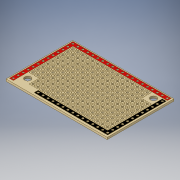
# Autodesk Inventor part: Proto Board
Saved by Autodesk Inventor 2016 (Build 200138000, 138)
## iProperties
Created: 2015-11-30
Part Number: Proto Board
Material: Generic
Document SubType Name: Modeling
Designer: Spooner
Density: 1 g/cm^3
Appearance: Beige
Author: Spooner
Autodesk Inventor part; units mm, degrees
(part 1 of 2)
ref_plane "YZ Plane" through (0, 0, 0) normal (1, 0, 0) x (0, 1, 0)
ref_plane "XZ Plane" through (0, 0, 0) normal (0, 1, 0) x (-1, 0, 0)
ref_plane "XY Plane" through (0, 0, 0) normal (0, 0, 1) x (1, 0, 0)
sketch "Sketch1" plane through (0, 0, 0) normal (0, 1, 0) x (-1, 0, 0)
  line L0 (0, 0) -> (-51.7271, 0)
  line L1 (-51.7271, 0) -> (-51.7271, -34.1376)
  line L2 (-51.7271, -34.1376) -> (0, -34.1376)
  line L3 (0, -34.1376) -> (0, 0)
  circle A0 centre (-5.3848, -5.7023) radius 1.524
  circle A1 centre (-46.3423, -29.0957) radius 1.524
  dimension "d0" = 51.7271
  dimension "d1" = 34.1376
  dimension "d2" = 3.8608
  dimension "d3" = 3.8608
  dimension "d4" = 3.5179
  dimension "d5" = 4.1783
  dimension "d6" = 3.048
  constraints: 8 end point, 2 centre point, 2 parallel, 1 equal radius, 1 horizontal, 1 perpendicular
  measures "d0" distance of L1.end L2.end
  measures "d1" distance of L2.end L0.start
  measures "d2" distance edge to line of A0 L3
  measures "d3" distance edge to line of A1 L1
  measures "d4" distance edge to line of A1 L2
  measures "d5" distance edge to line of A0 L0
  measures "d6" diameter of A0
extrude "Extrusion1" add sketch "Sketch1" along normal blind 1.016
sketch "Sketch2" plane through (0, 1.016, 0) normal (0, 1, 0) x (1, 0, 0)
  circle A0 centre (1.5494, 2.159) radius 0.508
  line L0 (0, 0) -> (51.7271, 0) projected
  line L1 (0, 34.1376) -> (0, 0) projected
  dimension "d9" = 1.016
  dimension "d10" = 1.651
  dimension "d11" = 1.0414
  constraints: 1 centre point
  measures "d9" diameter of A0
  measures "d10" distance edge to line of A0 L0
  measures "d11" distance edge to line of A0 L1
extrude "Extrusion2" cut sketch "Sketch2" against normal through all
sketch "Sketch6" plane through (0, 1.016, 0) normal (0, 1, 0) x (1, 0, 0)
  circle A0 centre (1.5494, 2.159) radius 0.508 projected
  line L0 (2.5654, 1.143) -> (0.5334, 1.143)
  line L1 (0.5334, 1.143) -> (0.5334, 3.175)
  line L2 (0.5334, 3.175) -> (2.5654, 3.175)
  line L3 (2.5654, 3.175) -> (2.5654, 1.143)
  line L4 (2.5654, 1.143) -> (0.5334, 3.175) construction
  line L5 (0.5334, 1.143) -> (2.5654, 3.175) construction
  point P0 (0, 0)
  dimension "d30" = 2.032
  constraints: 12 end point, 2 midpoint, 2 parallel, 2 perpendicular, 1 horizontal
  measures "d30" distance of L1.end L2.end
extrude "Extrusion6" add sketch "Sketch6" along normal blind 0.0254
pattern_linear "Rectangular Pattern1" count 13 spacing 2.54 along (0, 0, -1) count 20 spacing 2.54 along (1, 0, 0) of "Extrusion2", "Extrusion6"
sketch "Sketch7" plane through (0, 1.016, 0) normal (0, 1, 0) x (1, 0, 0)
  line L0 (5.6134, 3.683) -> (7.6454, 3.683) projected
  line L1 (3.0734, 8.255) -> (7.6454, 8.255)
  line L2 (7.6454, 8.255) -> (7.6454, 3.683)
  line L3 (7.6454, 3.683) -> (3.0734, 3.683)
  line L4 (3.0734, 3.683) -> (3.0734, 8.255)
  line L5 (5.1054, 3.175) -> (3.0734, 3.175) projected
  line L6 (10.6934, 1.143) -> (12.7254, 1.143) projected
  line L7 (3.0734, 3.175) -> (12.7254, 3.175)
  line L8 (12.7254, 3.175) -> (12.7254, 1.143)
  line L9 (12.7254, 1.143) -> (3.0734, 1.143)
  line L10 (3.0734, 1.143) -> (3.0734, 3.175)
  line L11 (45.7454, 31.115) -> (43.7134, 31.115) projected
  line L12 (43.7134, 31.115) -> (48.2854, 31.115)
  line L13 (48.2854, 31.115) -> (48.2854, 26.543)
  line L14 (48.2854, 26.543) -> (43.7134, 26.543)
  line L15 (43.7134, 26.543) -> (43.7134, 31.115)
  point P0 (0, 0)
  constraints: 24 end point, 6 parallel, 3 horizontal, 3 perpendicular, 2 coincident
extrude "Extrusion7" cut sketch "Sketch7" along normal blind 0.0254
sketch "Sketch8" plane through (0, 1.016, 0) normal (0, 1, 0) x (1, 0, 0)
  line L0 (3.2284, 8.3049) -> (7.6265, 8.3049)
  line L1 (7.6265, 8.3049) -> (7.6265, 3.6729)
  line L2 (7.6265, 3.6729) -> (3.2284, 3.6729)
  line L3 (3.2284, 3.6729) -> (3.2284, 8.3049)
  line L4 (3.2284, 3.1582) -> (12.6328, 3.1582)
  line L5 (12.6328, 3.1582) -> (12.6328, 1.0527)
  line L6 (12.6328, 1.0527) -> (3.2284, 1.0527)
  line L7 (3.2284, 1.0527) -> (3.2284, 3.1582)
  circle A0 centre (5.3848, 5.7023) radius 1.524
  arc A1 (6.1798, 7.0025) -> (4.5048, 6.9465) centre (5.3848, 5.7023) ccw projected
  circle A2 centre (46.3423, 29.0957) radius 1.524
  arc A3 (47.4393, 28.0378) -> (47.6879, 29.8111) centre (46.3423, 29.0957) ccw projected
  line L8 (43.7779, 31.0602) -> (48.4629, 31.0602)
  line L9 (48.4629, 31.0602) -> (48.4629, 26.515)
  line L10 (48.4629, 26.515) -> (43.7779, 26.515)
  line L11 (43.7779, 26.515) -> (43.7779, 31.0602)
  point P0 (0, 0)
  constraints: 24 end point, 6 parallel, 3 horizontal, 3 perpendicular, 1 point on line, 8 other
extrude "Extrusion8" add sketch "Sketch8" against normal up to surface (1.016 mm away)
sketch "Sketch9" plane through (0, 1.016, 0) normal (0, 1, 0) x (1, 0, 0)
  circle A0 centre (1.5494, 2.159) radius 0.508 projected
  line L0 (0.5334, 1.143) -> (2.5654, 1.143) projected
  line L1 (2.5654, 1.143) -> (2.5654, 3.175) projected
  line L2 (2.5654, 3.175) -> (0.5334, 3.175) projected
  line L3 (0.5334, 3.175) -> (0.5334, 1.143) projected
  circle A1 centre (5.3848, 5.7023) radius 1.524 projected
  circle A2 centre (46.3423, 29.0957) radius 1.524 projected
  line L4 (48.7934, 31.623) -> (48.7934, 33.655) projected
  line L5 (48.7934, 33.655) -> (50.8254, 33.655) projected
  line L6 (50.8254, 33.655) -> (50.8254, 31.623) projected
  line L7 (50.8254, 31.623) -> (48.7934, 31.623) projected
  line L8 (48.7934, 29.083) -> (48.7934, 31.115) projected
  line L9 (48.7934, 31.115) -> (50.8254, 31.115) projected
  line L10 (50.8254, 31.115) -> (50.8254, 29.083) projected
  line L11 (50.8254, 29.083) -> (48.7934, 29.083) projected
  line L12 (48.7934, 26.543) -> (48.7934, 28.575) projected
  line L13 (48.7934, 28.575) -> (50.8254, 28.575) projected
  line L14 (50.8254, 28.575) -> (50.8254, 26.543) projected
  line L15 (50.8254, 26.543) -> (48.7934, 26.543) projected
  line L16 (48.7934, 24.003) -> (48.7934, 26.035) projected
  line L17 (48.7934, 26.035) -> (50.8254, 26.035) projected
  line L18 (50.8254, 26.035) -> (50.8254, 24.003) projected
  line L19 (50.8254, 24.003) -> (48.7934, 24.003) projected
  line L20 (48.7934, 21.463) -> (48.7934, 23.495) projected
  line L21 (48.7934, 23.495) -> (50.8254, 23.495) projected
  line L22 (50.8254, 23.495) -> (50.8254, 21.463) projected
  line L23 (50.8254, 21.463) -> (48.7934, 21.463) projected
  line L24 (48.7934, 18.923) -> (48.7934, 20.955) projected
  line L25 (48.7934, 20.955) -> (50.8254, 20.955) projected
  line L26 (50.8254, 20.955) -> (50.8254, 18.923) projected
  line L27 (50.8254, 18.923) -> (48.7934, 18.923) projected
  line L28 (48.7934, 16.383) -> (48.7934, 18.415) projected
  line L29 (48.7934, 18.415) -> (50.8254, 18.415) projected
  line L30 (50.8254, 18.415) -> (50.8254, 16.383) projected
  line L31 (50.8254, 16.383) -> (48.7934, 16.383) projected
  line L32 (48.7934, 13.843) -> (48.7934, 15.875) projected
  line L33 (48.7934, 15.875) -> (50.8254, 15.875) projected
  line L34 (50.8254, 15.875) -> (50.8254, 13.843) projected
  line L35 (50.8254, 13.843) -> (48.7934, 13.843) projected
  line L36 (48.7934, 11.303) -> (48.7934, 13.335) projected
  line L37 (48.7934, 13.335) -> (50.8254, 13.335) projected
  line L38 (50.8254, 13.335) -> (50.8254, 11.303) projected
  line L39 (50.8254, 11.303) -> (48.7934, 11.303) projected
  line L40 (48.7934, 8.763) -> (48.7934, 10.795) projected
  line L41 (48.7934, 10.795) -> (50.8254, 10.795) projected
  line L42 (50.8254, 10.795) -> (50.8254, 8.763) projected
  line L43 (50.8254, 8.763) -> (48.7934, 8.763) projected
  line L44 (48.7934, 6.223) -> (48.7934, 8.255) projected
  line L45 (48.7934, 8.255) -> (50.8254, 8.255) projected
  line L46 (50.8254, 8.255) -> (50.8254, 6.223) projected
  line L47 (50.8254, 6.223) -> (48.7934, 6.223) projected
  line L48 (48.7934, 3.683) -> (48.7934, 5.715) projected
  line L49 (48.7934, 5.715) -> (50.8254, 5.715) projected
  line L50 (50.8254, 5.715) -> (50.8254, 3.683) projected
  line L51 (50.8254, 3.683) -> (48.7934, 3.683) projected
  line L52 (48.7934, 1.143) -> (48.7934, 3.175) projected
  line L53 (48.7934, 3.175) -> (50.8254, 3.175) projected
  line L54 (50.8254, 3.175) -> (50.8254, 1.143) projected
  line L55 (50.8254, 1.143) -> (48.7934, 1.143) projected
  line L56 (46.2534, 31.623) -> (46.2534, 33.655) projected
  line L57 (46.2534, 33.655) -> (48.2854, 33.655) projected
  line L58 (48.2854, 33.655) -> (48.2854, 31.623) projected
  line L59 (48.2854, 31.623) -> (46.2534, 31.623) projected
  line L60 (46.2534, 24.003) -> (46.2534, 26.035) projected
  line L61 (46.2534, 26.035) -> (48.2854, 26.035) projected
  line L62 (48.2854, 26.035) -> (48.2854, 24.003) projected
  line L63 (48.2854, 24.003) -> (46.2534, 24.003) projected
  line L64 (46.2534, 21.463) -> (46.2534, 23.495) projected
  line L65 (46.2534, 23.495) -> (48.2854, 23.495) projected
  line L66 (48.2854, 23.495) -> (48.2854, 21.463) projected
  line L67 (48.2854, 21.463) -> (46.2534, 21.463) projected
  line L68 (46.2534, 18.923) -> (46.2534, 20.955) projected
  line L69 (46.2534, 20.955) -> (48.2854, 20.955) projected
  line L70 (48.2854, 20.955) -> (48.2854, 18.923) projected
  line L71 (48.2854, 18.923) -> (46.2534, 18.923) projected
  line L72 (46.2534, 16.383) -> (46.2534, 18.415) projected
  line L73 (46.2534, 18.415) -> (48.2854, 18.415) projected
  line L74 (48.2854, 18.415) -> (48.2854, 16.383) projected
  line L75 (48.2854, 16.383) -> (46.2534, 16.383) projected
  line L76 (46.2534, 13.843) -> (46.2534, 15.875) projected
  line L77 (46.2534, 15.875) -> (48.2854, 15.875) projected
  line L78 (48.2854, 15.875) -> (48.2854, 13.843) projected
  line L79 (48.2854, 13.843) -> (46.2534, 13.843) projected
  line L80 (46.2534, 11.303) -> (46.2534, 13.335) projected
  line L81 (46.2534, 13.335) -> (48.2854, 13.335) projected
  line L82 (48.2854, 13.335) -> (48.2854, 11.303) projected
  line L83 (48.2854, 11.303) -> (46.2534, 11.303) projected
  line L84 (46.2534, 8.763) -> (46.2534, 10.795) projected
  line L85 (46.2534, 10.795) -> (48.2854, 10.795) projected
  line L86 (48.2854, 10.795) -> (48.2854, 8.763) projected
  line L87 (48.2854, 8.763) -> (46.2534, 8.763) projected
  line L88 (46.2534, 6.223) -> (46.2534, 8.255) projected
  line L89 (46.2534, 8.255) -> (48.2854, 8.255) projected
  line L90 (48.2854, 8.255) -> (48.2854, 6.223) projected
  line L91 (48.2854, 6.223) -> (46.2534, 6.223) projected
  line L92 (46.2534, 3.683) -> (46.2534, 5.715) projected
  line L93 (46.2534, 5.715) -> (48.2854, 5.715) projected
  line L94 (48.2854, 5.715) -> (48.2854, 3.683) projected
  line L95 (48.2854, 3.683) -> (46.2534, 3.683) projected
  line L96 (46.2534, 1.143) -> (46.2534, 3.175) projected
  line L97 (46.2534, 3.175) -> (48.2854, 3.175) projected
  line L98 (48.2854, 3.175) -> (48.2854, 1.143) projected
  line L99 (48.2854, 1.143) -> (46.2534, 1.143) projected
  line L100 (43.7134, 31.623) -> (43.7134, 33.655) projected
  line L101 (43.7134, 33.655) -> (45.7454, 33.655) projected
  line L102 (45.7454, 33.655) -> (45.7454, 31.623) projected
  line L103 (45.7454, 31.623) -> (43.7134, 31.623) projected
  line L104 (43.7134, 24.003) -> (43.7134, 26.035) projected
  line L105 (43.7134, 26.035) -> (45.7454, 26.035) projected
  line L106 (45.7454, 26.035) -> (45.7454, 24.003) projected
  line L107 (45.7454, 24.003) -> (43.7134, 24.003) projected
  line L108 (43.7134, 21.463) -> (43.7134, 23.495) projected
  line L109 (43.7134, 23.495) -> (45.7454, 23.495) projected
  line L110 (45.7454, 23.495) -> (45.7454, 21.463) projected
  line L111 (45.7454, 21.463) -> (43.7134, 21.463) projected
  line L112 (43.7134, 18.923) -> (43.7134, 20.955) projected
  line L113 (43.7134, 20.955) -> (45.7454, 20.955) projected
  line L114 (45.7454, 20.955) -> (45.7454, 18.923) projected
  line L115 (45.7454, 18.923) -> (43.7134, 18.923) projected
  line L116 (43.7134, 16.383) -> (43.7134, 18.415) projected
  line L117 (43.7134, 18.415) -> (45.7454, 18.415) projected
  line L118 (45.7454, 18.415) -> (45.7454, 16.383) projected
  line L119 (45.7454, 16.383) -> (43.7134, 16.383) projected
  line L120 (43.7134, 13.843) -> (43.7134, 15.875) projected
  line L121 (43.7134, 15.875) -> (45.7454, 15.875) projected
  line L122 (45.7454, 15.875) -> (45.7454, 13.843) projected
  line L123 (45.7454, 13.843) -> (43.7134, 13.843) projected
  line L124 (43.7134, 11.303) -> (43.7134, 13.335) projected
  line L125 (43.7134, 13.335) -> (45.7454, 13.335) projected
  line L126 (45.7454, 13.335) -> (45.7454, 11.303) projected
  line L127 (45.7454, 11.303) -> (43.7134, 11.303) projected
  line L128 (43.7134, 8.763) -> (43.7134, 10.795) projected
  line L129 (43.7134, 10.795) -> (45.7454, 10.795) projected
  line L130 (45.7454, 10.795) -> (45.7454, 8.763) projected
  line L131 (45.7454, 8.763) -> (43.7134, 8.763) projected
  line L132 (43.7134, 6.223) -> (43.7134, 8.255) projected
  line L133 (43.7134, 8.255) -> (45.7454, 8.255) projected
  line L134 (45.7454, 8.255) -> (45.7454, 6.223) projected
  line L135 (45.7454, 6.223) -> (43.7134, 6.223) projected
  line L136 (43.7134, 3.683) -> (43.7134, 5.715) projected
  line L137 (43.7134, 5.715) -> (45.7454, 5.715) projected
  line L138 (45.7454, 5.715) -> (45.7454, 3.683) projected
  line L139 (45.7454, 3.683) -> (43.7134, 3.683) projected
  line L140 (43.7134, 1.143) -> (43.7134, 3.175) projected
  line L141 (43.7134, 3.175) -> (45.7454, 3.175) projected
  line L142 (45.7454, 3.175) -> (45.7454, 1.143) projected
  line L143 (45.7454, 1.143) -> (43.7134, 1.143) projected
  line L144 (41.1734, 31.623) -> (41.1734, 33.655) projected
  line L145 (41.1734, 33.655) -> (43.2054, 33.655) projected
  line L146 (43.2054, 33.655) -> (43.2054, 31.623) projected
  line L147 (43.2054, 31.623) -> (41.1734, 31.623) projected
  line L148 (41.1734, 29.083) -> (41.1734, 31.115) projected
  line L149 (41.1734, 31.115) -> (43.2054, 31.115) projected
  line L150 (43.2054, 31.115) -> (43.2054, 29.083) projected
  line L151 (43.2054, 29.083) -> (41.1734, 29.083) projected
  line L152 (41.1734, 26.543) -> (41.1734, 28.575) projected
  line L153 (41.1734, 28.575) -> (43.2054, 28.575) projected
  line L154 (43.2054, 28.575) -> (43.2054, 26.543) projected
  line L155 (43.2054, 26.543) -> (41.1734, 26.543) projected
  line L156 (41.1734, 24.003) -> (41.1734, 26.035) projected
  line L157 (41.1734, 26.035) -> (43.2054, 26.035) projected
  line L158 (43.2054, 26.035) -> (43.2054, 24.003) projected
  line L159 (43.2054, 24.003) -> (41.1734, 24.003) projected
  line L160 (41.1734, 21.463) -> (41.1734, 23.495) projected
  line L161 (41.1734, 23.495) -> (43.2054, 23.495) projected
  line L162 (43.2054, 23.495) -> (43.2054, 21.463) projected
  line L163 (43.2054, 21.463) -> (41.1734, 21.463) projected
  line L164 (41.1734, 18.923) -> (41.1734, 20.955) projected
  line L165 (41.1734, 20.955) -> (43.2054, 20.955) projected
  line L166 (43.2054, 20.955) -> (43.2054, 18.923) projected
  line L167 (43.2054, 18.923) -> (41.1734, 18.923) projected
  line L168 (41.1734, 16.383) -> (41.1734, 18.415) projected
  line L169 (41.1734, 18.415) -> (43.2054, 18.415) projected
  line L170 (43.2054, 18.415) -> (43.2054, 16.383) projected
  line L171 (43.2054, 16.383) -> (41.1734, 16.383) projected
  line L172 (41.1734, 13.843) -> (41.1734, 15.875) projected
  line L173 (41.1734, 15.875) -> (43.2054, 15.875) projected
  line L174 (43.2054, 15.875) -> (43.2054, 13.843) projected
  line L175 (43.2054, 13.843) -> (41.1734, 13.843) projected
  line L176 (41.1734, 11.303) -> (41.1734, 13.335) projected
  line L177 (41.1734, 13.335) -> (43.2054, 13.335) projected
  line L178 (43.2054, 13.335) -> (43.2054, 11.303) projected
  line L179 (43.2054, 11.303) -> (41.1734, 11.303) projected
  line L180 (41.1734, 8.763) -> (41.1734, 10.795) projected
  line L181 (41.1734, 10.795) -> (43.2054, 10.795) projected
  line L182 (43.2054, 10.795) -> (43.2054, 8.763) projected
  line L183 (43.2054, 8.763) -> (41.1734, 8.763) projected
  line L184 (41.1734, 6.223) -> (41.1734, 8.255) projected
  line L185 (41.1734, 8.255) -> (43.2054, 8.255) projected
  line L186 (43.2054, 8.255) -> (43.2054, 6.223) projected
  line L187 (43.2054, 6.223) -> (41.1734, 6.223) projected
  line L188 (41.1734, 3.683) -> (41.1734, 5.715) projected
  line L189 (41.1734, 5.715) -> (43.2054, 5.715) projected
  line L190 (43.2054, 5.715) -> (43.2054, 3.683) projected
  line L191 (43.2054, 3.683) -> (41.1734, 3.683) projected
  line L192 (41.1734, 1.143) -> (41.1734, 3.175) projected
  line L193 (41.1734, 3.175) -> (43.2054, 3.175) projected
  line L194 (43.2054, 3.175) -> (43.2054, 1.143) projected
  line L195 (43.2054, 1.143) -> (41.1734, 1.143) projected
  line L196 (38.6334, 31.623) -> (38.6334, 33.655) projected
  line L197 (38.6334, 33.655) -> (40.6654, 33.655) projected
  line L198 (40.6654, 33.655) -> (40.6654, 31.623) projected
  line L199 (40.6654, 31.623) -> (38.6334, 31.623) projected
  line L200 (38.6334, 29.083) -> (38.6334, 31.115) projected
  line L201 (38.6334, 31.115) -> (40.6654, 31.115) projected
  line L202 (40.6654, 31.115) -> (40.6654, 29.083) projected
  line L203 (40.6654, 29.083) -> (38.6334, 29.083) projected
  line L204 (38.6334, 26.543) -> (38.6334, 28.575) projected
  line L205 (38.6334, 28.575) -> (40.6654, 28.575) projected
  line L206 (40.6654, 28.575) -> (40.6654, 26.543) projected
  line L207 (40.6654, 26.543) -> (38.6334, 26.543) projected
  line L208 (38.6334, 24.003) -> (38.6334, 26.035) projected
  line L209 (38.6334, 26.035) -> (40.6654, 26.035) projected
  line L210 (40.6654, 26.035) -> (40.6654, 24.003) projected
  line L211 (40.6654, 24.003) -> (38.6334, 24.003) projected
  line L212 (38.6334, 21.463) -> (38.6334, 23.495) projected
  line L213 (38.6334, 23.495) -> (40.6654, 23.495) projected
  line L214 (40.6654, 23.495) -> (40.6654, 21.463) projected
  line L215 (40.6654, 21.463) -> (38.6334, 21.463) projected
  line L216 (38.6334, 18.923) -> (38.6334, 20.955) projected
  line L217 (38.6334, 20.955) -> (40.6654, 20.955) projected
  line L218 (40.6654, 20.955) -> (40.6654, 18.923) projected
  line L219 (40.6654, 18.923) -> (38.6334, 18.923) projected
  line L220 (38.6334, 16.383) -> (38.6334, 18.415) projected
  line L221 (38.6334, 18.415) -> (40.6654, 18.415) projected
  line L222 (40.6654, 18.415) -> (40.6654, 16.383) projected
  line L223 (40.6654, 16.383) -> (38.6334, 16.383) projected
  line L224 (38.6334, 13.843) -> (38.6334, 15.875) projected
  line L225 (38.6334, 15.875) -> (40.6654, 15.875) projected
  line L226 (40.6654, 15.875) -> (40.6654, 13.843) projected
  line L227 (40.6654, 13.843) -> (38.6334, 13.843) projected
  line L228 (38.6334, 11.303) -> (38.6334, 13.335) projected
  line L229 (38.6334, 13.335) -> (40.6654, 13.335) projected
  line L230 (40.6654, 13.335) -> (40.6654, 11.303) projected
  line L231 (40.6654, 11.303) -> (38.6334, 11.303) projected
  line L232 (38.6334, 8.763) -> (38.6334, 10.795) projected
  line L233 (38.6334, 10.795) -> (40.6654, 10.795) projected
  line L234 (40.6654, 10.795) -> (40.6654, 8.763) projected
  line L235 (40.6654, 8.763) -> (38.6334, 8.763) projected
  line L236 (38.6334, 6.223) -> (38.6334, 8.255) projected
  line L237 (38.6334, 8.255) -> (40.6654, 8.255) projected
  line L238 (40.6654, 8.255) -> (40.6654, 6.223) projected
  line L239 (40.6654, 6.223) -> (38.6334, 6.223) projected
  line L240 (38.6334, 3.683) -> (38.6334, 5.715) projected
  line L241 (38.6334, 5.715) -> (40.6654, 5.715) projected
  line L242 (40.6654, 5.715) -> (40.6654, 3.683) projected
  line L243 (40.6654, 3.683) -> (38.6334, 3.683) projected
  line L244 (38.6334, 1.143) -> (38.6334, 3.175) projected
  line L245 (38.6334, 3.175) -> (40.6654, 3.175) projected
  line L246 (40.6654, 3.175) -> (40.6654, 1.143) projected
  line L247 (40.6654, 1.143) -> (38.6334, 1.143) projected
  line L248 (36.0934, 31.623) -> (36.0934, 33.655) projected
  line L249 (36.0934, 33.655) -> (38.1254, 33.655) projected
  line L250 (38.1254, 33.655) -> (38.1254, 31.623) projected
  line L251 (38.1254, 31.623) -> (36.0934, 31.623) projected
  line L252 (36.0934, 29.083) -> (36.0934, 31.115) projected
  line L253 (36.0934, 31.115) -> (38.1254, 31.115) projected
  line L254 (38.1254, 31.115) -> (38.1254, 29.083) projected
  line L255 (38.1254, 29.083) -> (36.0934, 29.083) projected
  line L256 (36.0934, 26.543) -> (36.0934, 28.575) projected
  line L257 (36.0934, 28.575) -> (38.1254, 28.575) projected
  line L258 (38.1254, 28.575) -> (38.1254, 26.543) projected
  line L259 (38.1254, 26.543) -> (36.0934, 26.543) projected
  line L260 (36.0934, 24.003) -> (36.0934, 26.035) projected
  line L261 (36.0934, 26.035) -> (38.1254, 26.035) projected
  line L262 (38.1254, 26.035) -> (38.1254, 24.003) projected
  line L263 (38.1254, 24.003) -> (36.0934, 24.003) projected
  line L264 (36.0934, 21.463) -> (36.0934, 23.495) projected
  line L265 (36.0934, 23.495) -> (38.1254, 23.495) projected
  line L266 (38.1254, 23.495) -> (38.1254, 21.463) projected
  line L267 (38.1254, 21.463) -> (36.0934, 21.463) projected
  line L268 (36.0934, 18.923) -> (36.0934, 20.955) projected
  line L269 (36.0934, 20.955) -> (38.1254, 20.955) projected
  line L270 (38.1254, 20.955) -> (38.1254, 18.923) projected
  line L271 (38.1254, 18.923) -> (36.0934, 18.923) projected
  line L272 (36.0934, 16.383) -> (36.0934, 18.415) projected
  line L273 (36.0934, 18.415) -> (38.1254, 18.415) projected
  line L274 (38.1254, 18.415) -> (38.1254, 16.383) projected
  line L275 (38.1254, 16.383) -> (36.0934, 16.383) projected
  line L276 (36.0934, 13.843) -> (36.0934, 15.875) projected
  line L277 (36.0934, 15.875) -> (38.1254, 15.875) projected
  line L278 (38.1254, 15.875) -> (38.1254, 13.843) projected
  line L279 (38.1254, 13.843) -> (36.0934, 13.843) projected
  line L280 (36.0934, 11.303) -> (36.0934, 13.335) projected
  line L281 (36.0934, 13.335) -> (38.1254, 13.335) projected
  line L282 (38.1254, 13.335) -> (38.1254, 11.303) projected
  line L283 (38.1254, 11.303) -> (36.0934, 11.303) projected
  line L284 (36.0934, 8.763) -> (36.0934, 10.795) projected
  line L285 (36.0934, 10.795) -> (38.1254, 10.795) projected
  line L286 (38.1254, 10.795) -> (38.1254, 8.763) projected
  line L287 (38.1254, 8.763) -> (36.0934, 8.763) projected
  line L288 (36.0934, 6.223) -> (36.0934, 8.255) projected
  line L289 (36.0934, 8.255) -> (38.1254, 8.255) projected
  line L290 (38.1254, 8.255) -> (38.1254, 6.223) projected
  line L291 (38.1254, 6.223) -> (36.0934, 6.223) projected
  line L292 (36.0934, 3.683) -> (36.0934, 5.715) projected
  line L293 (36.0934, 5.715) -> (38.1254, 5.715) projected
  line L294 (38.1254, 5.715) -> (38.1254, 3.683) projected
  line L295 (38.1254, 3.683) -> (36.0934, 3.683) projected
  line L296 (36.0934, 1.143) -> (36.0934, 3.175) projected
  line L297 (36.0934, 3.175) -> (38.1254, 3.175) projected
  line L298 (38.1254, 3.175) -> (38.1254, 1.143) projected
  line L299 (38.1254, 1.143) -> (36.0934, 1.143) projected
  line L300 (33.5534, 31.623) -> (33.5534, 33.655) projected
  line L301 (33.5534, 33.655) -> (35.5854, 33.655) projected
  line L302 (35.5854, 33.655) -> (35.5854, 31.623) projected
  line L303 (35.5854, 31.623) -> (33.5534, 31.623) projected
  line L304 (33.5534, 29.083) -> (33.5534, 31.115) projected
  line L305 (33.5534, 31.115) -> (35.5854, 31.115) projected
  line L306 (35.5854, 31.115) -> (35.5854, 29.083) projected
  line L307 (35.5854, 29.083) -> (33.5534, 29.083) projected
  line L308 (33.5534, 26.543) -> (33.5534, 28.575) projected
  line L309 (33.5534, 28.575) -> (35.5854, 28.575) projected
  line L310 (35.5854, 28.575) -> (35.5854, 26.543) projected
  line L311 (35.5854, 26.543) -> (33.5534, 26.543) projected
  line L312 (33.5534, 24.003) -> (33.5534, 26.035) projected
  line L313 (33.5534, 26.035) -> (35.5854, 26.035) projected
  line L314 (35.5854, 26.035) -> (35.5854, 24.003) projected
  line L315 (35.5854, 24.003) -> (33.5534, 24.003) projected
  line L316 (33.5534, 21.463) -> (33.5534, 23.495) projected
  line L317 (33.5534, 23.495) -> (35.5854, 23.495) projected
  line L318 (35.5854, 23.495) -> (35.5854, 21.463) projected
  line L319 (35.5854, 21.463) -> (33.5534, 21.463) projected
  line L320 (33.5534, 18.923) -> (33.5534, 20.955) projected
  line L321 (33.5534, 20.955) -> (35.5854, 20.955) projected
  line L322 (35.5854, 20.955) -> (35.5854, 18.923) projected
  line L323 (35.5854, 18.923) -> (33.5534, 18.923) projected
  line L324 (33.5534, 16.383) -> (33.5534, 18.415) projected
  line L325 (33.5534, 18.415) -> (35.5854, 18.415) projected
  line L326 (35.5854, 18.415) -> (35.5854, 16.383) projected
  line L327 (35.5854, 16.383) -> (33.5534, 16.383) projected
  line L328 (33.5534, 13.843) -> (33.5534, 15.875) projected
  line L329 (33.5534, 15.875) -> (35.5854, 15.875) projected
  line L330 (35.5854, 15.875) -> (35.5854, 13.843) projected
  line L331 (35.5854, 13.843) -> (33.5534, 13.843) projected
  line L332 (33.5534, 11.303) -> (33.5534, 13.335) projected
  line L333 (33.5534, 13.335) -> (35.5854, 13.335) projected
  line L334 (35.5854, 13.335) -> (35.5854, 11.303) projected
  line L335 (35.5854, 11.303) -> (33.5534, 11.303) projected
  line L336 (33.5534, 8.763) -> (33.5534, 10.795) projected
  line L337 (33.5534, 10.795) -> (35.5854, 10.795) projected
  line L338 (35.5854, 10.795) -> (35.5854, 8.763) projected
  line L339 (35.5854, 8.763) -> (33.5534, 8.763) projected
  line L340 (33.5534, 6.223) -> (33.5534, 8.255) projected
  line L341 (33.5534, 8.255) -> (35.5854, 8.255) projected
  line L342 (35.5854, 8.255) -> (35.5854, 6.223) projected
  line L343 (35.5854, 6.223) -> (33.5534, 6.223) projected
  line L344 (33.5534, 3.683) -> (33.5534, 5.715) projected
  line L345 (33.5534, 5.715) -> (35.5854, 5.715) projected
  line L346 (35.5854, 5.715) -> (35.5854, 3.683) projected
  line L347 (35.5854, 3.683) -> (33.5534, 3.683) projected
  line L348 (33.5534, 1.143) -> (33.5534, 3.175) projected
  line L349 (33.5534, 3.175) -> (35.5854, 3.175) projected
  line L350 (35.5854, 3.175) -> (35.5854, 1.143) projected
  line L351 (35.5854, 1.143) -> (33.5534, 1.143) projected
  line L352 (31.0134, 31.623) -> (31.0134, 33.655) projected
  line L353 (31.0134, 33.655) -> (33.0454, 33.655) projected
  line L354 (33.0454, 33.655) -> (33.0454, 31.623) projected
  line L355 (33.0454, 31.623) -> (31.0134, 31.623) projected
  line L356 (31.0134, 29.083) -> (31.0134, 31.115) projected
  line L357 (31.0134, 31.115) -> (33.0454, 31.115) projected
  line L358 (33.0454, 31.115) -> (33.0454, 29.083) projected
  line L359 (33.0454, 29.083) -> (31.0134, 29.083) projected
  line L360 (31.0134, 26.543) -> (31.0134, 28.575) projected
  line L361 (31.0134, 28.575) -> (33.0454, 28.575) projected
  line L362 (33.0454, 28.575) -> (33.0454, 26.543) projected
  line L363 (33.0454, 26.543) -> (31.0134, 26.543) projected
  line L364 (31.0134, 24.003) -> (31.0134, 26.035) projected
  line L365 (31.0134, 26.035) -> (33.0454, 26.035) projected
  line L366 (33.0454, 26.035) -> (33.0454, 24.003) projected
  line L367 (33.0454, 24.003) -> (31.0134, 24.003) projected
  line L368 (31.0134, 21.463) -> (31.0134, 23.495) projected
  line L369 (31.0134, 23.495) -> (33.0454, 23.495) projected
  line L370 (33.0454, 23.495) -> (33.0454, 21.463) projected
  line L371 (33.0454, 21.463) -> (31.0134, 21.463) projected
  line L372 (31.0134, 18.923) -> (31.0134, 20.955) projected
  line L373 (31.0134, 20.955) -> (33.0454, 20.955) projected
  line L374 (33.0454, 20.955) -> (33.0454, 18.923) projected
  line L375 (33.0454, 18.923) -> (31.0134, 18.923) projected
  line L376 (31.0134, 16.383) -> (31.0134, 18.415) projected
  line L377 (31.0134, 18.415) -> (33.0454, 18.415) projected
  line L378 (33.0454, 18.415) -> (33.0454, 16.383) projected
  line L379 (33.0454, 16.383) -> (31.0134, 16.383) projected
  line L380 (31.0134, 13.843) -> (31.0134, 15.875) projected
  line L381 (31.0134, 15.875) -> (33.0454, 15.875) projected
  line L382 (33.0454, 15.875) -> (33.0454, 13.843) projected
  line L383 (33.0454, 13.843) -> (31.0134, 13.843) projected
  line L384 (31.0134, 11.303) -> (31.0134, 13.335) projected
  line L385 (31.0134, 13.335) -> (33.0454, 13.335) projected
  line L386 (33.0454, 13.335) -> (33.0454, 11.303) projected
  line L387 (33.0454, 11.303) -> (31.0134, 11.303) projected
  line L388 (31.0134, 8.763) -> (31.0134, 10.795) projected
  line L389 (31.0134, 10.795) -> (33.0454, 10.795) projected
  line L390 (33.0454, 10.795) -> (33.0454, 8.763) projected
  line L391 (33.0454, 8.763) -> (31.0134, 8.763) projected
  line L392 (31.0134, 6.223) -> (31.0134, 8.255) projected
  line L393 (31.0134, 8.255) -> (33.0454, 8.255) projected
  line L394 (33.0454, 8.255) -> (33.0454, 6.223) projected
  line L395 (33.0454, 6.223) -> (31.0134, 6.223) projected
  line L396 (31.0134, 3.683) -> (31.0134, 5.715) projected
  line L397 (31.0134, 5.715) -> (33.0454, 5.715) projected
  line L398 (33.0454, 5.715) -> (33.0454, 3.683) projected
  line L399 (33.0454, 3.683) -> (31.0134, 3.683) projected
  line L400 (31.0134, 1.143) -> (31.0134, 3.175) projected
  line L401 (31.0134, 3.175) -> (33.0454, 3.175) projected
  line L402 (33.0454, 3.175) -> (33.0454, 1.143) projected
  line L403 (33.0454, 1.143) -> (31.0134, 1.143) projected
  line L404 (28.4734, 31.623) -> (28.4734, 33.655) projected
  line L405 (28.4734, 33.655) -> (30.5054, 33.655) projected
  line L406 (30.5054, 33.655) -> (30.5054, 31.623) projected
  line L407 (30.5054, 31.623) -> (28.4734, 31.623) projected
  line L408 (28.4734, 29.083) -> (28.4734, 31.115) projected
  line L409 (28.4734, 31.115) -> (30.5054, 31.115) projected
  line L410 (30.5054, 31.115) -> (30.5054, 29.083) projected
  line L411 (30.5054, 29.083) -> (28.4734, 29.083) projected
  line L412 (28.4734, 26.543) -> (28.4734, 28.575) projected
  line L413 (28.4734, 28.575) -> (30.5054, 28.575) projected
  line L414 (30.5054, 28.575) -> (30.5054, 26.543) projected
  line L415 (30.5054, 26.543) -> (28.4734, 26.543) projected
  line L416 (28.4734, 24.003) -> (28.4734, 26.035) projected
  line L417 (28.4734, 26.035) -> (30.5054, 26.035) projected
  line L418 (30.5054, 26.035) -> (30.5054, 24.003) projected
  line L419 (30.5054, 24.003) -> (28.4734, 24.003) projected
  line L420 (28.4734, 21.463) -> (28.4734, 23.495) projected
  line L421 (28.4734, 23.495) -> (30.5054, 23.495) projected
  line L422 (30.5054, 23.495) -> (30.5054, 21.463) projected
  line L423 (30.5054, 21.463) -> (28.4734, 21.463) projected
  line L424 (28.4734, 18.923) -> (28.4734, 20.955) projected
  line L425 (28.4734, 20.955) -> (30.5054, 20.955) projected
  line L426 (30.5054, 20.955) -> (30.5054, 18.923) projected
  line L427 (30.5054, 18.923) -> (28.4734, 18.923) projected
  line L428 (28.4734, 16.383) -> (28.4734, 18.415) projected
  line L429 (28.4734, 18.415) -> (30.5054, 18.415) projected
  line L430 (30.5054, 18.415) -> (30.5054, 16.383) projected
  line L431 (30.5054, 16.383) -> (28.4734, 16.383) projected
  line L432 (28.4734, 13.843) -> (28.4734, 15.875) projected
  line L433 (28.4734, 15.875) -> (30.5054, 15.875) projected
  line L434 (30.5054, 15.875) -> (30.5054, 13.843) projected
  line L435 (30.5054, 13.843) -> (28.4734, 13.843) projected
  line L436 (28.4734, 11.303) -> (28.4734, 13.335) projected
  line L437 (28.4734, 13.335) -> (30.5054, 13.335) projected
  line L438 (30.5054, 13.335) -> (30.5054, 11.303) projected
  line L439 (30.5054, 11.303) -> (28.4734, 11.303) projected
  line L440 (28.4734, 8.763) -> (28.4734, 10.795) projected
  line L441 (28.4734, 10.795) -> (30.5054, 10.795) projected
  line L442 (30.5054, 10.795) -> (30.5054, 8.763) projected
  line L443 (30.5054, 8.763) -> (28.4734, 8.763) projected
  line L444 (28.4734, 6.223) -> (28.4734, 8.255) projected
  line L445 (28.4734, 8.255) -> (30.5054, 8.255) projected
  line L446 (30.5054, 8.255) -> (30.5054, 6.223) projected
  line L447 (30.5054, 6.223) -> (28.4734, 6.223) projected
  line L448 (28.4734, 3.683) -> (28.4734, 5.715) projected
  line L449 (28.4734, 5.715) -> (30.5054, 5.715) projected
  line L450 (30.5054, 5.715) -> (30.5054, 3.683) projected
  line L451 (30.5054, 3.683) -> (28.4734, 3.683) projected
  line L452 (28.4734, 1.143) -> (28.4734, 3.175) projected
  line L453 (28.4734, 3.175) -> (30.5054, 3.175) projected
  line L454 (30.5054, 3.175) -> (30.5054, 1.143) projected
  line L455 (30.5054, 1.143) -> (28.4734, 1.143) projected
  line L456 (25.9334, 31.623) -> (25.9334, 33.655) projected
  line L457 (25.9334, 33.655) -> (27.9654, 33.655) projected
  line L458 (27.9654, 33.655) -> (27.9654, 31.623) projected
  line L459 (27.9654, 31.623) -> (25.9334, 31.623) projected
  line L460 (25.9334, 29.083) -> (25.9334, 31.115) projected
  line L461 (25.9334, 31.115) -> (27.9654, 31.115) projected
  line L462 (27.9654, 31.115) -> (27.9654, 29.083) projected
  line L463 (27.9654, 29.083) -> (25.9334, 29.083) projected
  line L464 (25.9334, 26.543) -> (25.9334, 28.575) projected
  line L465 (25.9334, 28.575) -> (27.9654, 28.575) projected
  line L466 (27.9654, 28.575) -> (27.9654, 26.543) projected
  line L467 (27.9654, 26.543) -> (25.9334, 26.543) projected
  line L468 (25.9334, 24.003) -> (25.9334, 26.035) projected
  line L469 (25.9334, 26.035) -> (27.9654, 26.035) projected
  line L470 (27.9654, 26.035) -> (27.9654, 24.003) projected
  line L471 (27.9654, 24.003) -> (25.9334, 24.003) projected
  line L472 (25.9334, 21.463) -> (25.9334, 23.495) projected
  line L473 (25.9334, 23.495) -> (27.9654, 23.495) projected
  line L474 (27.9654, 23.495) -> (27.9654, 21.463) projected
  line L475 (27.9654, 21.463) -> (25.9334, 21.463) projected
  line L476 (25.9334, 18.923) -> (25.9334, 20.955) projected
  line L477 (25.9334, 20.955) -> (27.9654, 20.955) projected
  line L478 (27.9654, 20.955) -> (27.9654, 18.923) projected
  line L479 (27.9654, 18.923) -> (25.9334, 18.923) projected
  line L480 (25.9334, 16.383) -> (25.9334, 18.415) projected
  line L481 (25.9334, 18.415) -> (27.9654, 18.415) projected
  line L482 (27.9654, 18.415) -> (27.9654, 16.383) projected
  line L483 (27.9654, 16.383) -> (25.9334, 16.383) projected
  line L484 (25.9334, 13.843) -> (25.9334, 15.875) projected
  line L485 (25.9334, 15.875) -> (27.9654, 15.875) projected
  line L486 (27.9654, 15.875) -> (27.9654, 13.843) projected
  line L487 (27.9654, 13.843) -> (25.9334, 13.843) projected
  line L488 (25.9334, 11.303) -> (25.9334, 13.335) projected
  line L489 (25.9334, 13.335) -> (27.9654, 13.335) projected
  line L490 (27.9654, 13.335) -> (27.9654, 11.303) projected
  line L491 (27.9654, 11.303) -> (25.9334, 11.303) projected
  line L492 (25.9334, 8.763) -> (25.9334, 10.795) projected
  line L493 (25.9334, 10.795) -> (27.9654, 10.795) projected
  line L494 (27.9654, 10.795) -> (27.9654, 8.763) projected
  line L495 (27.9654, 8.763) -> (25.9334, 8.763) projected
  line L496 (25.9334, 6.223) -> (25.9334, 8.255) projected
  line L497 (25.9334, 8.255) -> (27.9654, 8.255) projected
  line L498 (27.9654, 8.255) -> (27.9654, 6.223) projected
  line L499 (27.9654, 6.223) -> (25.9334, 6.223) projected
  line L500 (25.9334, 3.683) -> (25.9334, 5.715) projected
  line L501 (25.9334, 5.715) -> (27.9654, 5.715) projected
  line L502 (27.9654, 5.715) -> (27.9654, 3.683) projected
  line L503 (27.9654, 3.683) -> (25.9334, 3.683) projected
  line L504 (25.9334, 1.143) -> (25.9334, 3.175) projected
  line L505 (25.9334, 3.175) -> (27.9654, 3.175) projected
  line L506 (27.9654, 3.175) -> (27.9654, 1.143) projected
  line L507 (27.9654, 1.143) -> (25.9334, 1.143) projected
  line L508 (23.3934, 31.623) -> (23.3934, 33.655) projected
  line L509 (23.3934, 33.655) -> (25.4254, 33.655) projected
  line L510 (25.4254, 33.655) -> (25.4254, 31.623) projected
  line L511 (25.4254, 31.623) -> (23.3934, 31.623) projected
  line L512 (23.3934, 29.083) -> (23.3934, 31.115) projected
  line L513 (23.3934, 31.115) -> (25.4254, 31.115) projected
  line L514 (25.4254, 31.115) -> (25.4254, 29.083) projected
  line L515 (25.4254, 29.083) -> (23.3934, 29.083) projected
  line L516 (23.3934, 26.543) -> (23.3934, 28.575) projected
  line L517 (23.3934, 28.575) -> (25.4254, 28.575) projected
  line L518 (25.4254, 28.575) -> (25.4254, 26.543) projected
  line L519 (25.4254, 26.543) -> (23.3934, 26.543) projected
  line L520 (23.3934, 24.003) -> (23.3934, 26.035) projected
  line L521 (23.3934, 26.035) -> (25.4254, 26.035) projected
  line L522 (25.4254, 26.035) -> (25.4254, 24.003) projected
  line L523 (25.4254, 24.003) -> (23.3934, 24.003) projected
  line L524 (23.3934, 21.463) -> (23.3934, 23.495) projected
  line L525 (23.3934, 23.495) -> (25.4254, 23.495) projected
  line L526 (25.4254, 23.495) -> (25.4254, 21.463) projected
  line L527 (25.4254, 21.463) -> (23.3934, 21.463) projected
  line L528 (23.3934, 18.923) -> (23.3934, 20.955) projected
  line L529 (23.3934, 20.955) -> (25.4254, 20.955) projected
  line L530 (25.4254, 20.955) -> (25.4254, 18.923) projected
  line L531 (25.4254, 18.923) -> (23.3934, 18.923) projected
  line L532 (23.3934, 16.383) -> (23.3934, 18.415) projected
  line L533 (23.3934, 18.415) -> (25.4254, 18.415) projected
  line L534 (25.4254, 18.415) -> (25.4254, 16.383) projected
  line L535 (25.4254, 16.383) -> (23.3934, 16.383) projected
  line L536 (23.3934, 13.843) -> (23.3934, 15.875) projected
  line L537 (23.3934, 15.875) -> (25.4254, 15.875) projected
  line L538 (25.4254, 15.875) -> (25.4254, 13.843) projected
  line L539 (25.4254, 13.843) -> (23.3934, 13.843) projected
  line L540 (23.3934, 11.303) -> (23.3934, 13.335) projected
  line L541 (23.3934, 13.335) -> (25.4254, 13.335) projected
  line L542 (25.4254, 13.335) -> (25.4254, 11.303) projected
  line L543 (25.4254, 11.303) -> (23.3934, 11.303) projected
  line L544 (23.3934, 8.763) -> (23.3934, 10.795) projected
  line L545 (23.3934, 10.795) -> (25.4254, 10.795) projected
  line L546 (25.4254, 10.795) -> (25.4254, 8.763) projected
  line L547 (25.4254, 8.763) -> (23.3934, 8.763) projected
  line L548 (23.3934, 6.223) -> (23.3934, 8.255) projected
  line L549 (23.3934, 8.255) -> (25.4254, 8.255) projected
  line L550 (25.4254, 8.255) -> (25.4254, 6.223) projected
  line L551 (25.4254, 6.223) -> (23.3934, 6.223) projected
  line L552 (23.3934, 3.683) -> (23.3934, 5.715) projected
  line L553 (23.3934, 5.715) -> (25.4254, 5.715) projected
  line L554 (25.4254, 5.715) -> (25.4254, 3.683) projected
  line L555 (25.4254, 3.683) -> (23.3934, 3.683) projected
  line L556 (23.3934, 1.143) -> (23.3934, 3.175) projected
  line L557 (23.3934, 3.175) -> (25.4254, 3.175) projected
  line L558 (25.4254, 3.175) -> (25.4254, 1.143) projected
  line L559 (25.4254, 1.143) -> (23.3934, 1.143) projected
  line L560 (20.8534, 31.623) -> (20.8534, 33.655) projected
  line L561 (20.8534, 33.655) -> (22.8854, 33.655) projected
  line L562 (22.8854, 33.655) -> (22.8854, 31.623) projected
  line L563 (22.8854, 31.623) -> (20.8534, 31.623) projected
  line L564 (20.8534, 29.083) -> (20.8534, 31.115) projected
  line L565 (20.8534, 31.115) -> (22.8854, 31.115) projected
  line L566 (22.8854, 31.115) -> (22.8854, 29.083) projected
  line L567 (22.8854, 29.083) -> (20.8534, 29.083) projected
  line L568 (20.8534, 26.543) -> (20.8534, 28.575) projected
  line L569 (20.8534, 28.575) -> (22.8854, 28.575) projected
  line L570 (22.8854, 28.575) -> (22.8854, 26.543) projected
  line L571 (22.8854, 26.543) -> (20.8534, 26.543) projected
  line L572 (20.8534, 24.003) -> (20.8534, 26.035) projected
  line L573 (20.8534, 26.035) -> (22.8854, 26.035) projected
  line L574 (22.8854, 26.035) -> (22.8854, 24.003) projected
  line L575 (22.8854, 24.003) -> (20.8534, 24.003) projected
  line L576 (20.8534, 21.463) -> (20.8534, 23.495) projected
  line L577 (20.8534, 23.495) -> (22.8854, 23.495) projected
  line L578 (22.8854, 23.495) -> (22.8854, 21.463) projected
  line L579 (22.8854, 21.463) -> (20.8534, 21.463) projected
  line L580 (20.8534, 18.923) -> (20.8534, 20.955) projected
  line L581 (20.8534, 20.955) -> (22.8854, 20.955) projected
  line L582 (22.8854, 20.955) -> (22.8854, 18.923) projected
  line L583 (22.8854, 18.923) -> (20.8534, 18.923) projected
  line L584 (20.8534, 16.383) -> (20.8534, 18.415) projected
  line L585 (20.8534, 18.415) -> (22.8854, 18.415) projected
  line L586 (22.8854, 18.415) -> (22.8854, 16.383) projected
  line L587 (22.8854, 16.383) -> (20.8534, 16.383) projected
  line L588 (20.8534, 13.843) -> (20.8534, 15.875) projected
  line L589 (20.8534, 15.875) -> (22.8854, 15.875) projected
  line L590 (22.8854, 15.875) -> (22.8854, 13.843) projected
  line L591 (22.8854, 13.843) -> (20.8534, 13.843) projected
  line L592 (20.8534, 11.303) -> (20.8534, 13.335) projected
  line L593 (20.8534, 13.335) -> (22.8854, 13.335) projected
  line L594 (22.8854, 13.335) -> (22.8854, 11.303) projected
  line L595 (22.8854, 11.303) -> (20.8534, 11.303) projected
  line L596 (20.8534, 8.763) -> (20.8534, 10.795) projected
  line L597 (20.8534, 10.795) -> (22.8854, 10.795) projected
  line L598 (22.8854, 10.795) -> (22.8854, 8.763) projected
  line L599 (22.8854, 8.763) -> (20.8534, 8.763) projected
  line L600 (20.8534, 6.223) -> (20.8534, 8.255) projected
  line L601 (20.8534, 8.255) -> (22.8854, 8.255) projected
  line L602 (22.8854, 8.255) -> (22.8854, 6.223) projected
  line L603 (22.8854, 6.223) -> (20.8534, 6.223) projected
  line L604 (20.8534, 3.683) -> (20.8534, 5.715) projected
  line L605 (20.8534, 5.715) -> (22.8854, 5.715) projected
  line L606 (22.8854, 5.715) -> (22.8854, 3.683) projected
  line L607 (22.8854, 3.683) -> (20.8534, 3.683) projected
  line L608 (20.8534, 1.143) -> (20.8534, 3.175) projected
  line L609 (20.8534, 3.175) -> (22.8854, 3.175) projected
  line L610 (22.8854, 3.175) -> (22.8854, 1.143) projected
  line L611 (22.8854, 1.143) -> (20.8534, 1.143) projected
  line L612 (18.3134, 31.623) -> (18.3134, 33.655) projected
  line L613 (18.3134, 33.655) -> (20.3454, 33.655) projected
  line L614 (20.3454, 33.655) -> (20.3454, 31.623) projected
  line L615 (20.3454, 31.623) -> (18.3134, 31.623) projected
  line L616 (18.3134, 29.083) -> (18.3134, 31.115) projected
  line L617 (18.3134, 31.115) -> (20.3454, 31.115) projected
  line L618 (20.3454, 31.115) -> (20.3454, 29.083) projected
  line L619 (20.3454, 29.083) -> (18.3134, 29.083) projected
  line L620 (18.3134, 26.543) -> (18.3134, 28.575) projected
  line L621 (18.3134, 28.575) -> (20.3454, 28.575) projected
  line L622 (20.3454, 28.575) -> (20.3454, 26.543) projected
  line L623 (20.3454, 26.543) -> (18.3134, 26.543) projected
  line L624 (18.3134, 24.003) -> (18.3134, 26.035) projected
  line L625 (18.3134, 26.035) -> (20.3454, 26.035) projected
  line L626 (20.3454, 26.035) -> (20.3454, 24.003) projected
  line L627 (20.3454, 24.003) -> (18.3134, 24.003) projected
  line L628 (18.3134, 21.463) -> (18.3134, 23.495) projected
  line L629 (18.3134, 23.495) -> (20.3454, 23.495) projected
  line L630 (20.3454, 23.495) -> (20.3454, 21.463) projected
  line L631 (20.3454, 21.463) -> (18.3134, 21.463) projected
  line L632 (18.3134, 18.923) -> (18.3134, 20.955) projected
  line L633 (18.3134, 20.955) -> (20.3454, 20.955) projected
  line L634 (20.3454, 20.955) -> (20.3454, 18.923) projected
  line L635 (20.3454, 18.923) -> (18.3134, 18.923) projected
  line L636 (18.3134, 16.383) -> (18.3134, 18.415) projected
  line L637 (18.3134, 18.415) -> (20.3454, 18.415) projected
  line L638 (20.3454, 18.415) -> (20.3454, 16.383) projected
  line L639 (20.3454, 16.383) -> (18.3134, 16.383) projected
  line L640 (18.3134, 13.843) -> (18.3134, 15.875) projected
  line L641 (18.3134, 15.875) -> (20.3454, 15.875) projected
  line L642 (20.3454, 15.875) -> (20.3454, 13.843) projected
  line L643 (20.3454, 13.843) -> (18.3134, 13.843) projected
  line L644 (18.3134, 11.303) -> (18.3134, 13.335) projected
  line L645 (18.3134, 13.335) -> (20.3454, 13.335) projected
  line L646 (20.3454, 13.335) -> (20.3454, 11.303) projected
  line L647 (20.3454, 11.303) -> (18.3134, 11.303) projected
  line L648 (18.3134, 8.763) -> (18.3134, 10.795) projected
  line L649 (18.3134, 10.795) -> (20.3454, 10.795) projected
  line L650 (20.3454, 10.795) -> (20.3454, 8.763) projected
  line L651 (20.3454, 8.763) -> (18.3134, 8.763) projected
  line L652 (18.3134, 6.223) -> (18.3134, 8.255) projected
  line L653 (18.3134, 8.255) -> (20.3454, 8.255) projected
  line L654 (20.3454, 8.255) -> (20.3454, 6.223) projected
  line L655 (20.3454, 6.223) -> (18.3134, 6.223) projected
  line L656 (18.3134, 3.683) -> (18.3134, 5.715) projected
  line L657 (18.3134, 5.715) -> (20.3454, 5.715) projected
  line L658 (20.3454, 5.715) -> (20.3454, 3.683) projected
  line L659 (20.3454, 3.683) -> (18.3134, 3.683) projected
  line L660 (18.3134, 1.143) -> (18.3134, 3.175) projected
  line L661 (18.3134, 3.175) -> (20.3454, 3.175) projected
  line L662 (20.3454, 3.175) -> (20.3454, 1.143) projected
  line L663 (20.3454, 1.143) -> (18.3134, 1.143) projected
  line L664 (15.7734, 31.623) -> (15.7734, 33.655) projected
  line L665 (15.7734, 33.655) -> (17.8054, 33.655) projected
  line L666 (17.8054, 33.655) -> (17.8054, 31.623) projected
  line L667 (17.8054, 31.623) -> (15.7734, 31.623) projected
  line L668 (15.7734, 29.083) -> (15.7734, 31.115) projected
  line L669 (15.7734, 31.115) -> (17.8054, 31.115) projected
  line L670 (17.8054, 31.115) -> (17.8054, 29.083) projected
  line L671 (17.8054, 29.083) -> (15.7734, 29.083) projected
  line L672 (15.7734, 26.543) -> (15.7734, 28.575) projected
  line L673 (15.7734, 28.575) -> (17.8054, 28.575) projected
  line L674 (17.8054, 28.575) -> (17.8054, 26.543) projected
  line L675 (17.8054, 26.543) -> (15.7734, 26.543) projected
  line L676 (15.7734, 24.003) -> (15.7734, 26.035) projected
  line L677 (15.7734, 26.035) -> (17.8054, 26.035) projected
  line L678 (17.8054, 26.035) -> (17.8054, 24.003) projected
  line L679 (17.8054, 24.003) -> (15.7734, 24.003) projected
  line L680 (15.7734, 21.463) -> (15.7734, 23.495) projected
  line L681 (15.7734, 23.495) -> (17.8054, 23.495) projected
  line L682 (17.8054, 23.495) -> (17.8054, 21.463) projected
  line L683 (17.8054, 21.463) -> (15.7734, 21.463) projected
  line L684 (15.7734, 18.923) -> (15.7734, 20.955) projected
  line L685 (15.7734, 20.955) -> (17.8054, 20.955) projected
  line L686 (17.8054, 20.955) -> (17.8054, 18.923) projected
  line L687 (17.8054, 18.923) -> (15.7734, 18.923) projected
  line L688 (15.7734, 16.383) -> (15.7734, 18.415) projected
  line L689 (15.7734, 18.415) -> (17.8054, 18.415) projected
  line L690 (17.8054, 18.415) -> (17.8054, 16.383) projected
  line L691 (17.8054, 16.383) -> (15.7734, 16.383) projected
  line L692 (15.7734, 13.843) -> (15.7734, 15.875) projected
  line L693 (15.7734, 15.875) -> (17.8054, 15.875) projected
  line L694 (17.8054, 15.875) -> (17.8054, 13.843) projected
  line L695 (17.8054, 13.843) -> (15.7734, 13.843) projected
  line L696 (15.7734, 11.303) -> (15.7734, 13.335) projected
  line L697 (15.7734, 13.335) -> (17.8054, 13.335) projected
  line L698 (17.8054, 13.335) -> (17.8054, 11.303) projected
  line L699 (17.8054, 11.303) -> (15.7734, 11.303) projected
  line L700 (15.7734, 8.763) -> (15.7734, 10.795) projected
  line L701 (15.7734, 10.795) -> (17.8054, 10.795) projected
  line L702 (17.8054, 10.795) -> (17.8054, 8.763) projected
  line L703 (17.8054, 8.763) -> (15.7734, 8.763) projected
  line L704 (15.7734, 6.223) -> (15.7734, 8.255) projected
  line L705 (15.7734, 8.255) -> (17.8054, 8.255) projected
  line L706 (17.8054, 8.255) -> (17.8054, 6.223) projected
  line L707 (17.8054, 6.223) -> (15.7734, 6.223) projected
  line L708 (15.7734, 3.683) -> (15.7734, 5.715) projected
  line L709 (15.7734, 5.715) -> (17.8054, 5.715) projected
  line L710 (17.8054, 5.715) -> (17.8054, 3.683) projected
  line L711 (17.8054, 3.683) -> (15.7734, 3.683) projected
  line L712 (15.7734, 1.143) -> (15.7734, 3.175) projected
  line L713 (15.7734, 3.175) -> (17.8054, 3.175) projected
  line L714 (17.8054, 3.175) -> (17.8054, 1.143) projected
  line L715 (17.8054, 1.143) -> (15.7734, 1.143) projected
  line L716 (13.2334, 31.623) -> (13.2334, 33.655) projected
  line L717 (13.2334, 33.655) -> (15.2654, 33.655) projected
  line L718 (15.2654, 33.655) -> (15.2654, 31.623) projected
  line L719 (15.2654, 31.623) -> (13.2334, 31.623) projected
  line L720 (13.2334, 29.083) -> (13.2334, 31.115) projected
  line L721 (13.2334, 31.115) -> (15.2654, 31.115) projected
  line L722 (15.2654, 31.115) -> (15.2654, 29.083) projected
  line L723 (15.2654, 29.083) -> (13.2334, 29.083) projected
  line L724 (13.2334, 26.543) -> (13.2334, 28.575) projected
  line L725 (13.2334, 28.575) -> (15.2654, 28.575) projected
  line L726 (15.2654, 28.575) -> (15.2654, 26.543) projected
  line L727 (15.2654, 26.543) -> (13.2334, 26.543) projected
  line L728 (13.2334, 24.003) -> (13.2334, 26.035) projected
  line L729 (13.2334, 26.035) -> (15.2654, 26.035) projected
  line L730 (15.2654, 26.035) -> (15.2654, 24.003) projected
  line L731 (15.2654, 24.003) -> (13.2334, 24.003) projected
  line L732 (13.2334, 21.463) -> (13.2334, 23.495) projected
  line L733 (13.2334, 23.495) -> (15.2654, 23.495) projected
  line L734 (15.2654, 23.495) -> (15.2654, 21.463) projected
  line L735 (15.2654, 21.463) -> (13.2334, 21.463) projected
  line L736 (13.2334, 18.923) -> (13.2334, 20.955) projected
  line L737 (13.2334, 20.955) -> (15.2654, 20.955) projected
  line L738 (15.2654, 20.955) -> (15.2654, 18.923) projected
  line L739 (15.2654, 18.923) -> (13.2334, 18.923) projected
  line L740 (13.2334, 16.383) -> (13.2334, 18.415) projected
  line L741 (13.2334, 18.415) -> (15.2654, 18.415) projected
  line L742 (15.2654, 18.415) -> (15.2654, 16.383) projected
  line L743 (15.2654, 16.383) -> (13.2334, 16.383) projected
  line L744 (13.2334, 13.843) -> (13.2334, 15.875) projected
  line L745 (13.2334, 15.875) -> (15.2654, 15.875) projected
  line L746 (15.2654, 15.875) -> (15.2654, 13.843) projected
  line L747 (15.2654, 13.843) -> (13.2334, 13.843) projected
  line L748 (13.2334, 11.303) -> (13.2334, 13.335) projected
  line L749 (13.2334, 13.335) -> (15.2654, 13.335) projected
  line L750 (15.2654, 13.335) -> (15.2654, 11.303) projected
  line L751 (15.2654, 11.303) -> (13.2334, 11.303) projected
  line L752 (13.2334, 8.763) -> (13.2334, 10.795) projected
  line L753 (13.2334, 10.795) -> (15.2654, 10.795) projected
  line L754 (15.2654, 10.795) -> (15.2654, 8.763) projected
  line L755 (15.2654, 8.763) -> (13.2334, 8.763) projected
  line L756 (13.2334, 6.223) -> (13.2334, 8.255) projected
  line L757 (13.2334, 8.255) -> (15.2654, 8.255) projected
  line L758 (15.2654, 8.255) -> (15.2654, 6.223) projected
  line L759 (15.2654, 6.223) -> (13.2334, 6.223) projected
  line L760 (13.2334, 3.683) -> (13.2334, 5.715) projected
  line L761 (13.2334, 5.715) -> (15.2654, 5.715) projected
  line L762 (15.2654, 5.715) -> (15.2654, 3.683) projected
  line L763 (15.2654, 3.683) -> (13.2334, 3.683) projected
  line L764 (13.2334, 1.143) -> (13.2334, 3.175) projected
  line L765 (13.2334, 3.175) -> (15.2654, 3.175) projected
  line L766 (15.2654, 3.175) -> (15.2654, 1.143) projected
  line L767 (15.2654, 1.143) -> (13.2334, 1.143) projected
  line L768 (10.6934, 31.623) -> (10.6934, 33.655) projected
  line L769 (10.6934, 33.655) -> (12.7254, 33.655) projected
  line L770 (12.7254, 33.655) -> (12.7254, 31.623) projected
  line L771 (12.7254, 31.623) -> (10.6934, 31.623) projected
  line L772 (10.6934, 29.083) -> (10.6934, 31.115) projected
  line L773 (10.6934, 31.115) -> (12.7254, 31.115) projected
  line L774 (12.7254, 31.115) -> (12.7254, 29.083) projected
  line L775 (12.7254, 29.083) -> (10.6934, 29.083) projected
  line L776 (10.6934, 26.543) -> (10.6934, 28.575) projected
  line L777 (10.6934, 28.575) -> (12.7254, 28.575) projected
  line L778 (12.7254, 28.575) -> (12.7254, 26.543) projected
  line L779 (12.7254, 26.543) -> (10.6934, 26.543) projected
  line L780 (10.6934, 24.003) -> (10.6934, 26.035) projected
  line L781 (10.6934, 26.035) -> (12.7254, 26.035) projected
  line L782 (12.7254, 26.035) -> (12.7254, 24.003) projected
  line L783 (12.7254, 24.003) -> (10.6934, 24.003) projected
  line L784 (10.6934, 21.463) -> (10.6934, 23.495) projected
  line L785 (10.6934, 23.495) -> (12.7254, 23.495) projected
  line L786 (12.7254, 23.495) -> (12.7254, 21.463) projected
  line L787 (12.7254, 21.463) -> (10.6934, 21.463) projected
  line L788 (10.6934, 18.923) -> (10.6934, 20.955) projected
  line L789 (10.6934, 20.955) -> (12.7254, 20.955) projected
  line L790 (12.7254, 20.955) -> (12.7254, 18.923) projected
  line L791 (12.7254, 18.923) -> (10.6934, 18.923) projected
  line L792 (10.6934, 16.383) -> (10.6934, 18.415) projected
  line L793 (10.6934, 18.415) -> (12.7254, 18.415) projected
  line L794 (12.7254, 18.415) -> (12.7254, 16.383) projected
  line L795 (12.7254, 16.383) -> (10.6934, 16.383) projected
  line L796 (10.6934, 13.843) -> (10.6934, 15.875) projected
  line L797 (10.6934, 15.875) -> (12.7254, 15.875) projected
  line L798 (12.7254, 15.875) -> (12.7254, 13.843) projected
  line L799 (12.7254, 13.843) -> (10.6934, 13.843) projected
  line L800 (10.6934, 11.303) -> (10.6934, 13.335) projected
  line L801 (10.6934, 13.335) -> (12.7254, 13.335) projected
  line L802 (12.7254, 13.335) -> (12.7254, 11.303) projected
  line L803 (12.7254, 11.303) -> (10.6934, 11.303) projected
  line L804 (10.6934, 8.763) -> (10.6934, 10.795) projected
  line L805 (10.6934, 10.795) -> (12.7254, 10.795) projected
  line L806 (12.7254, 10.795) -> (12.7254, 8.763) projected
  line L807 (12.7254, 8.763) -> (10.6934, 8.763) projected
  line L808 (10.6934, 6.223) -> (10.6934, 8.255) projected
  line L809 (10.6934, 8.255) -> (12.7254, 8.255) projected
  line L810 (12.7254, 8.255) -> (12.7254, 6.223) projected
  line L811 (12.7254, 6.223) -> (10.6934, 6.223) projected
  line L812 (10.6934, 3.683) -> (10.6934, 5.715) projected
  line L813 (10.6934, 5.715) -> (12.7254, 5.715) projected
  line L814 (12.7254, 5.715) -> (12.7254, 3.683) projected
  line L815 (12.7254, 3.683) -> (10.6934, 3.683) projected
  line L816 (8.1534, 31.623) -> (8.1534, 33.655) projected
  line L817 (8.1534, 33.655) -> (10.1854, 33.655) projected
  line L818 (10.1854, 33.655) -> (10.1854, 31.623) projected
  line L819 (10.1854, 31.623) -> (8.1534, 31.623) projected
  line L820 (8.1534, 29.083) -> (8.1534, 31.115) projected
  line L821 (8.1534, 31.115) -> (10.1854, 31.115) projected
  line L822 (10.1854, 31.115) -> (10.1854, 29.083) projected
  line L823 (10.1854, 29.083) -> (8.1534, 29.083) projected
  line L824 (8.1534, 26.543) -> (8.1534, 28.575) projected
  line L825 (8.1534, 28.575) -> (10.1854, 28.575) projected
  line L826 (10.1854, 28.575) -> (10.1854, 26.543) projected
  line L827 (10.1854, 26.543) -> (8.1534, 26.543) projected
  line L828 (8.1534, 24.003) -> (8.1534, 26.035) projected
  line L829 (8.1534, 26.035) -> (10.1854, 26.035) projected
  line L830 (10.1854, 26.035) -> (10.1854, 24.003) projected
  line L831 (10.1854, 24.003) -> (8.1534, 24.003) projected
  line L832 (8.1534, 21.463) -> (8.1534, 23.495) projected
  line L833 (8.1534, 23.495) -> (10.1854, 23.495) projected
  line L834 (10.1854, 23.495) -> (10.1854, 21.463) projected
  line L835 (10.1854, 21.463) -> (8.1534, 21.463) projected
  line L836 (8.1534, 18.923) -> (8.1534, 20.955) projected
  line L837 (8.1534, 20.955) -> (10.1854, 20.955) projected
  line L838 (10.1854, 20.955) -> (10.1854, 18.923) projected
  line L839 (10.1854, 18.923) -> (8.1534, 18.923) projected
  line L840 (8.1534, 16.383) -> (8.1534, 18.415) projected
  line L841 (8.1534, 18.415) -> (10.1854, 18.415) projected
  line L842 (10.1854, 18.415) -> (10.1854, 16.383) projected
  line L843 (10.1854, 16.383) -> (8.1534, 16.383) projected
  line L844 (8.1534, 13.843) -> (8.1534, 15.875) projected
  line L845 (8.1534, 15.875) -> (10.1854, 15.875) projected
  line L846 (10.1854, 15.875) -> (10.1854, 13.843) projected
  line L847 (10.1854, 13.843) -> (8.1534, 13.843) projected
  line L848 (8.1534, 11.303) -> (8.1534, 13.335) projected
  line L849 (8.1534, 13.335) -> (10.1854, 13.335) projected
  line L850 (10.1854, 13.335) -> (10.1854, 11.303) projected
  line L851 (10.1854, 11.303) -> (8.1534, 11.303) projected
  line L852 (8.1534, 8.763) -> (8.1534, 10.795) projected
  line L853 (8.1534, 10.795) -> (10.1854, 10.795) projected
  line L854 (10.1854, 10.795) -> (10.1854, 8.763) projected
  line L855 (10.1854, 8.763) -> (8.1534, 8.763) projected
  line L856 (8.1534, 6.223) -> (8.1534, 8.255) projected
  line L857 (8.1534, 8.255) -> (10.1854, 8.255) projected
  line L858 (10.1854, 8.255) -> (10.1854, 6.223) projected
  line L859 (10.1854, 6.223) -> (8.1534, 6.223) projected
  line L860 (8.1534, 3.683) -> (8.1534, 5.715) projected
  line L861 (8.1534, 5.715) -> (10.1854, 5.715) projected
  line L862 (10.1854, 5.715) -> (10.1854, 3.683) projected
  line L863 (10.1854, 3.683) -> (8.1534, 3.683) projected
  line L864 (5.6134, 31.623) -> (5.6134, 33.655) projected
  line L865 (5.6134, 33.655) -> (7.6454, 33.655) projected
  line L866 (7.6454, 33.655) -> (7.6454, 31.623) projected
  line L867 (7.6454, 31.623) -> (5.6134, 31.623) projected
  line L868 (5.6134, 29.083) -> (5.6134, 31.115) projected
  line L869 (5.6134, 31.115) -> (7.6454, 31.115) projected
  line L870 (7.6454, 31.115) -> (7.6454, 29.083) projected
  line L871 (7.6454, 29.083) -> (5.6134, 29.083) projected
  line L872 (5.6134, 26.543) -> (5.6134, 28.575) projected
  line L873 (5.6134, 28.575) -> (7.6454, 28.575) projected
  line L874 (7.6454, 28.575) -> (7.6454, 26.543) projected
  line L875 (7.6454, 26.543) -> (5.6134, 26.543) projected
  line L876 (5.6134, 24.003) -> (5.6134, 26.035) projected
  line L877 (5.6134, 26.035) -> (7.6454, 26.035) projected
  line L878 (7.6454, 26.035) -> (7.6454, 24.003) projected
  line L879 (7.6454, 24.003) -> (5.6134, 24.003) projected
  line L880 (5.6134, 21.463) -> (5.6134, 23.495) projected
  line L881 (5.6134, 23.495) -> (7.6454, 23.495) projected
  line L882 (7.6454, 23.495) -> (7.6454, 21.463) projected
  line L883 (7.6454, 21.463) -> (5.6134, 21.463) projected
  line L884 (5.6134, 18.923) -> (5.6134, 20.955) projected
  line L885 (5.6134, 20.955) -> (7.6454, 20.955) projected
  line L886 (7.6454, 20.955) -> (7.6454, 18.923) projected
  line L887 (7.6454, 18.923) -> (5.6134, 18.923) projected
  line L888 (5.6134, 16.383) -> (5.6134, 18.415) projected
  line L889 (5.6134, 18.415) -> (7.6454, 18.415) projected
  line L890 (7.6454, 18.415) -> (7.6454, 16.383) projected
  line L891 (7.6454, 16.383) -> (5.6134, 16.383) projected